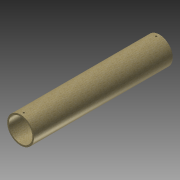
# Autodesk Inventor part: 8 ball paint roller
Saved by Autodesk Inventor 2012 (Build 160160000, 160)
## iProperties
Created: 2013-10-11
Part Number: 8 ball paint roller
Material: Default
Document SubType Name: Modeling
Designer: Bryce
Density: 1 g/cm^3
Author: Bryce
Autodesk Inventor part; units mm, degrees
ref_plane "YZ Plane" through (0, 0, 0) normal (1, 0, 0) x (0, 1, 0)
ref_plane "XZ Plane" through (0, 0, 0) normal (0, 1, 0) x (-1, 0, 0)
ref_plane "XY Plane" through (0, 0, 0) normal (0, 0, 1) x (1, 0, 0)
sketch "Sketch1" plane through (0, 0, 0) normal (0, 0, 1) x (1, 0, 0)
  circle A0 centre (0, 0) radius 26.9875
  circle A1 centre (0, 0) radius 23.8125
  dimension "d0" = 47.625
  dimension "d1" = 53.975
  constraints: 2 centre point, 2 coincident
  measures "d0" diameter of A1
  measures "d1" diameter of A0
extrude "Extrusion1" add sketch "Sketch1" along normal blind 279.4
sketch "Sketch2" plane through (0, 0, 0) normal (0, 1, 0) x (-1, 0, 0)
  line L0 (-26.9875, 0) -> (-26.9875, 279.4) projected
  line L1 (-26.9875, 0) -> (26.9875, 0) projected
  line L2 (26.9875, 0) -> (26.9875, 279.4) projected
  line L3 (-26.9875, 279.4) -> (26.9875, 279.4) projected
  circle A0 centre (0, 6.35) radius 1.7272
  circle A1 centre (0, 273.05) radius 1.7272
  point P0 (0, 0)
  point P1 (0, 279.4)
  point P2 (0, 0)
  dimension "d4" = 6.35
  dimension "d5" = 6.35
  dimension "d6" = 3.4544
  constraints: 2 centre point, 2 midpoint, 2 vertical alignment, 1 equal radius
  measures "d4" distance from line of L3 A1.centre
  measures "d5" distance of A0.centre point (0, 0)
  measures "d6" diameter of A1
extrude "Extrusion2" cut sketch "Sketch2" along normal through all contours A0 | A1
body "Solid1"
